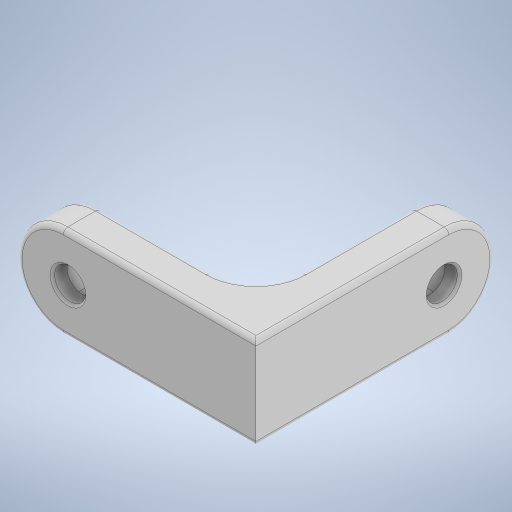
# Autodesk Inventor part: BoxBracket
Saved by Autodesk Inventor 2024.2 (Build 282272000, 272)
## iProperties
Created: 2023-11-15
Part Number: BoxBracket
Material: Generic
Document SubType Name: Modeling
Designer: Eric
Density: 1 g/cm^3
Appearance: Default
Author: Eric
Autodesk Inventor part; units mm, degrees
ref_plane "YZ Plane" through (0, 0, 0) normal (1, 0, 0) x (0, 1, 0)
ref_plane "XZ Plane" through (0, 0, 0) normal (0, 1, 0) x (-1, 0, 0)
ref_plane "XY Plane" through (0, 0, 0) normal (0, 0, 1) x (1, 0, 0)
sketch "Sketch1" plane through (0, 0, 0) normal (1, 0, 0) x (0, 1, 0)
  line L0 (0, 0) -> (10, 0)
  line L1 (10, 0) -> (10, -26)
  line L2 (10, -26) -> (0, -26)
  line L3 (0, -26) -> (0, 0)
  dimension "d0" = 10
  dimension "d1" = 26
  constraints: 8 end point, 2 parallel, 1 horizontal, 1 perpendicular
  measures "d0" distance of L1.end L2.end
  measures "d1" distance of L0.end L1.end
extrude "Extrusion1" add sketch "Sketch1" against normal blind 4
sketch "Sketch2" plane through (0, 0, 0) normal (0, 0, 1) x (1, 0, 0)
  line L0 (0, 0) -> (-4, 0) projected
  line L1 (0, 0) -> (-26, 0)
  line L2 (-26, 0) -> (-26, 10)
  line L3 (-26, 10) -> (0, 10)
  line L4 (0, 10) -> (0, 0)
  line L5 (0, 10) -> (0, 0) projected
  point P0 (-4, 0)
  dimension "d4" = 26
  constraints: 8 end point, 2 parallel, 1 collinear, 1 horizontal, 1 perpendicular
  measures "d4" distance of L2.end L3.end
extrude "Extrusion2" add sketch "Sketch2" against normal blind 4
sketch "Sketch3" plane through (-4, 0, 0) normal (-1, 0, 0) x (0, 0, 1)
  line L0 (-18.8546, 2.15) -> (-22.1454, 2.15)
  line L1 (-22.1454, 2.15) -> (-23.7909, 5)
  line L2 (-23.7909, 5) -> (-22.1454, 7.85)
  line L3 (-22.1454, 7.85) -> (-18.8546, 7.85)
  line L4 (-18.8546, 7.85) -> (-17.2091, 5)
  line L5 (-17.2091, 5) -> (-18.8546, 2.15)
  line L6 (-26, 10) -> (-26, 0) projected
  point P0 (0, 0)
  point P1 (-20.5, 5)
  point P2 (-26, 5)
  dimension "d7" = 5.7
  dimension "d8" = 5.5
  constraints: 12 end point, 1 horizontal, 1 horizontal alignment, 1 midpoint, 13 other
  measures "d7" distance between parallel lines of L0 L3
  measures "d8" distance from line of L6 point (-20.5, 5)
extrude "Extrusion3" cut sketch "Sketch3" against normal blind 2.4
sketch "Sketch4" plane through (-1.6, 0, 0) normal (-1, 0, 0) x (0, 0, 1)
  line L0 (-18.8546, 7.85) -> (-17.2091, 5) projected
  line L1 (-22.1454, 7.85) -> (-18.8546, 7.85) projected
  line L2 (-23.7909, 5) -> (-22.1454, 7.85) projected
  line L3 (-22.1454, 2.15) -> (-23.7909, 5) projected
  line L4 (-18.8546, 2.15) -> (-22.1454, 2.15) projected
  line L5 (-17.2091, 5) -> (-18.8546, 2.15) projected
  circle A0 centre (-20.5, 5) radius 1.7
  point P0 (0, 0)
  dimension "d11" = 3.4
  constraints: 1 centre point, 1 coincident
  measures "d11" diameter of A0
extrude "Extrusion4" cut sketch "Sketch4" against normal up to surface (1.6 mm away) contours A0
sketch "Sketch5" plane through (0, 0, -4) normal (0, 0, -1) x (-1, 0, 0)
  line L0 (22.1454, 2.15) -> (18.8546, 2.15)
  line L1 (18.8546, 2.15) -> (17.2091, 5)
  line L2 (17.2091, 5) -> (18.8546, 7.85)
  line L3 (18.8546, 7.85) -> (22.1454, 7.85)
  line L4 (22.1454, 7.85) -> (23.7909, 5)
  line L5 (23.7909, 5) -> (22.1454, 2.15)
  line L6 (26, 0) -> (26, 10) projected
  point P0 (0, 0)
  point P1 (20.5, 5)
  point P2 (26, 5)
  dimension "d14" = 5.7
  dimension "d15" = 5.5
  constraints: 12 end point, 1 horizontal, 1 horizontal alignment, 1 midpoint, 13 other
  measures "d14" distance between parallel lines of L3 L0
  measures "d15" distance from line of L6 point (20.5, 5)
extrude "Extrusion5" cut sketch "Sketch5" against normal blind 2.4
sketch "Sketch6" plane through (0, 0, -1.6) normal (0, 0, -1) x (-1, 0, 0)
  circle A0 centre (20.5, 5) radius 1.7
  point P0 (0, 0)
  dimension "d18" = 3.4
  constraints: 1 centre point, 1 coincident
  measures "d18" diameter of A0
extrude "Extrusion6" cut sketch "Sketch6" against normal up to surface (1.6 mm away)
fillet "Fillet1" radius 5 4 edges at (-2, 10, -26) (-2, 0, -26) (-26, 10, -2) (-26, 0, -2)
fillet "Fillet2" radius 5 1 edges at (-4, 5, -4)
fillet "Fillet3" radius 0.5 22 edges at (-4, 10, -15.0001) (-4, 8.5356, -24.5356) (-4, 5, -26) (-4, 1.4644, -24.5356) (-4, 0, -15.0001) (-5.4645, 0, -5.4645) (-15, 0, -4) (-24.5356, 8.5356, -4) (-26, 5, -4) (-24.5356, 1.4644, -4) (-15, 10, -4) (-5.4645, 10, -5.4645) (0, 1.4644, -24.5356) (0, 8.5356, -24.5356) (0, 5, -26) (0, 0, -10.5001) (0, 10, -10.5001) (-24.5356, 1.4644, 0) (-24.5356, 8.5356, 0) (-26, 5, 0) (-10.5, 0, 0) (-10.5, 10, 0)
chamfer "Chamfer1" distance 0.25 angle 45 2 edges at (0, 5, -22.2) (-18.8, 5, 0)
body "Solid1"
